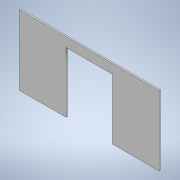
# Autodesk Inventor part: Vỏ F2
Saved by Autodesk Inventor 2020 (Build 240168000, 168)
## iProperties
Created: 2022-11-30
Part Number: Vỏ F2
Material: Generic
Document SubType Name: Modeling
Designer: ADMIN
Density: 1 g/cm^3
Appearance: Default
Author: ADMIN
Autodesk Inventor part; units mm, degrees
ref_plane "YZ Plane" through (0, 0, 0) normal (1, 0, 0) x (0, 1, 0)
ref_plane "XZ Plane" through (0, 0, 0) normal (0, 1, 0) x (-1, 0, 0)
ref_plane "XY Plane" through (0, 0, 0) normal (0, 0, 1) x (1, 0, 0)
sketch "Sketch1" plane through (0, 0, 0) normal (0, 0, 1) x (1, 0, 0)
  line L0 (300, 0) -> (300, 150)
  line L1 (300, 150) -> (0, 150)
  line L2 (0, 150) -> (0, 0)
  line L3 (200, 0) -> (200, 130)
  line L4 (200, 130) -> (100, 130)
  line L5 (100, 130) -> (100, 0)
  line L6 (0, 0) -> (100, 0)
  line L7 (200, 0) -> (300, 0)
  point P0 (150, 0)
  dimension "d0" = 300
  dimension "d1" = 150
  dimension "d2" = 100
  constraints: 16 end point, 4 parallel, 2 horizontal, 2 perpendicular
  measures "d0" distance of L1.end L0.end
  measures "d1" distance of L0.end L0.start
  measures "d2" distance of L4.end L3.end
extrude "Extrusion1" add sketch "Sketch1" along normal blind 3
body "Solid1"
